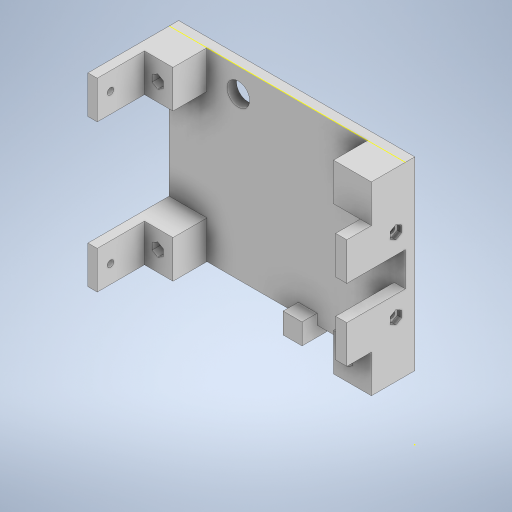
# Autodesk Inventor part: base-prototipo
Saved by Autodesk Inventor 2024.3 (Build 283343000, 343)
## iProperties
Created: 2025-10-16
Part Number: base-prototipo
Material: Genérico
Document SubType Name: Modeling
Designer: julio
Density: 1 g/cm^3
Appearance: Valor por defecto
Author: julio
## iProperties of the stored document Tapadera-prototipo_3DPrint.ipt
Created: 2025-10-16
Part Number: Tapadera-prototipo_3DPrint
Material: Genérico
Document SubType Name: Modeling
Designer: julio
Density: 1 g/cm^3
Appearance: Valor por defecto
Author: julio
Autodesk Inventor part; units mm, degrees
ref_plane "YZ Plane" through (0, 0, 0) normal (1, 0, 0) x (0, 1, 0)
ref_plane "XZ Plane" through (0, 0, 0) normal (0, 1, 0) x (-1, 0, 0)
ref_plane "XY Plane" through (0, 0, 0) normal (0, 0, 1) x (1, 0, 0)
sketch "Boceto1" plane through (0, 0, 0) normal (0, 0, 1) x (1, 0, 0)
  line L0 (-129.8713, 126.9415) -> (-4.8713, 126.9415)
  line L1 (-4.8713, 126.9415) -> (-4.8713, 28.9415)
  line L2 (-4.8713, 28.9415) -> (-129.8713, 28.9415)
  line L3 (-129.8713, 28.9415) -> (-129.8713, 126.9415)
  point P0 (0, 0)
  dimension "d0" = 98
  dimension "d1" = 125
  constraints: 8 end point, 2 parallel, 1 horizontal, 1 perpendicular
  measures "d0" distance of L0.end L1.end
  measures "d1" distance of L0.start L0.end
extrude "Extrusión1" add sketch "Boceto1" along normal blind 5
sketch "Boceto2" plane through (0, 0, 5) normal (0, 0, 1) x (1, 0, 0)
  line L0 (-4.8713, 126.9415) -> (-129.8713, 126.9415) projected
  point P0 (0, 0)
sketch "Boceto3" plane through (0, 0, 5) normal (0, 0, 1) x (1, 0, 0)
  line L0 (-129.8713, 126.9415) -> (-129.8713, 28.9415) projected
  line L1 (-124.9455, 121.4415) -> (-10.7713, 121.4415) construction
  line L2 (-10.7713, 121.4415) -> (-10.7713, 34.4465) construction
  line L3 (-10.7713, 34.4465) -> (-124.9455, 34.4465) construction
  line L4 (-124.9455, 34.4465) -> (-124.9455, 121.4415) construction
  line L5 (-4.8713, 28.9415) -> (-4.8713, 126.9415) projected
  line L6 (-4.8713, 126.9415) -> (-129.8713, 126.9415) projected
  line L7 (-129.8713, 28.9415) -> (-4.8713, 28.9415) projected
  line L8 (-129.8713, 126.9415) -> (-109.8713, 126.9415)
  line L9 (-109.8713, 126.9415) -> (-109.8713, 106.9415)
  line L10 (-109.8713, 106.9415) -> (-129.8713, 106.9415)
  line L11 (-129.8713, 106.9415) -> (-129.8713, 126.9415)
  line L12 (-129.8713, 28.9415) -> (-109.8713, 28.9415)
  line L13 (-109.8713, 28.9415) -> (-109.8713, 48.9415)
  line L14 (-109.8713, 48.9415) -> (-129.8713, 48.9415)
  line L15 (-129.8713, 48.9415) -> (-129.8713, 28.9415)
  line L16 (-4.8713, 28.9415) -> (-24.8713, 28.9415)
  line L17 (-24.8713, 28.9415) -> (-24.8713, 48.9415)
  line L18 (-24.8713, 48.9415) -> (-4.8713, 48.9415)
  line L19 (-4.8713, 48.9415) -> (-4.8713, 28.9415)
  line L20 (-4.8713, 126.9415) -> (-24.8713, 126.9415)
  line L21 (-24.8713, 126.9415) -> (-24.8713, 106.9415)
  line L22 (-24.8713, 106.9415) -> (-4.8713, 106.9415)
  line L23 (-4.8713, 106.9415) -> (-4.8713, 126.9415)
  point P0 (0, 0)
  point P1 (-109.8713, 28.9415)
  point P2 (-4.8713, 106.9415)
  dimension "d58" = 86.995
  dimension "d62" = 114.1741
  dimension "d67" = 5.9
  dimension "d68" = 4.9259
  dimension "d70" = 5.5
  dimension "d71" = 5.505
  dimension "d86" = 20
  dimension "d87" = 20
  dimension "d88" = 20
  dimension "d89" = 20
  dimension "d90" = 20
  dimension "d91" = 20
  dimension "d92" = 20
  dimension "d93" = 20
  constraints: 32 end point, 8 parallel, 4 horizontal, 4 perpendicular, 1 coincident, 2 other
  measures "d58" distance between parallel lines of L3 L1
  measures "d62" distance between parallel lines of L2 L4
  measures "d67" distance between parallel lines of L5 L2
  measures "d68" distance between parallel lines of L4 L0
  measures "d70" distance between parallel lines of L1 L6
  measures "d71" distance between parallel lines of L7 L3
  measures "d86" distance of L8.end L9.end
  measures "d87" distance of L9.end L10.end
  measures "d88" distance of L12.end L13.end
  measures "d89" distance of L13.end L14.end
  measures "d90" distance of L17.end L18.end
  measures "d91" distance of L16.end L17.end
  measures "d92" distance of L20.end L21.end
  measures "d93" distance of L21.end L22.end
extrude "Extrusión2" add sketch "Boceto3" along normal blind 18 contours L6 L9 L10 L0 | L14 L13 L7 L0 | L6 L5 L22 L21 | L17 L18 L5 L7
sketch "Boceto4" plane through (0, 0, 23) normal (0, 0, 1) x (1, 0, 0)
  line L0 (-124.9585, 121.4415) -> (-10.7843, 121.4415) construction
  line L1 (-10.7843, 121.4415) -> (-10.7843, 34.4465) construction
  line L2 (-10.7843, 34.4465) -> (-124.9585, 34.4465) construction
  line L3 (-124.9585, 34.4465) -> (-124.9585, 121.4415) construction
  line L4 (-4.8713, 48.9415) -> (-4.8713, 106.9415) projected
  line L5 (-24.8713, 126.9415) -> (-109.8713, 126.9415) projected
  line L6 (-109.8713, 28.9415) -> (-24.8713, 28.9415) projected
  line L7 (-129.8713, 106.9415) -> (-129.8713, 48.9415) projected
  line L8 (-129.8713, 106.9415) -> (-109.8713, 106.9415) projected
  line L9 (-129.8713, 126.9415) -> (-124.9585, 126.9415)
  line L10 (-124.9585, 126.9415) -> (-124.9585, 106.9415)
  line L11 (-124.9585, 106.9415) -> (-129.8713, 106.9415)
  line L12 (-129.8713, 106.9415) -> (-129.8713, 126.9415)
  line L13 (-124.9585, 28.9415) -> (-129.8713, 28.9415)
  line L14 (-129.8713, 28.9415) -> (-129.8713, 48.9415)
  line L15 (-129.8713, 48.9415) -> (-124.9585, 48.9415)
  line L16 (-124.9585, 48.9415) -> (-124.9585, 28.9415)
  line L17 (-4.8713, 28.9415) -> (-4.8713, 126.9415) projected
  point P0 (0, 0)
  point P1 (-10.7843, 48.9415)
  dimension "d105" = 5.5
  dimension "d106" = 5.505
  dimension "d108" = 5.913
  dimension "d109" = 4.9129
  dimension "d111" = 20
  constraints: 16 end point, 5 point on line, 4 parallel, 2 horizontal, 2 perpendicular, 2 other
  measures "d105" distance between parallel lines of L5 L0
  measures "d106" distance between parallel lines of L2 L6
  measures "d108" distance between parallel lines of L4 L1
  measures "d109" distance between parallel lines of L7 L3
  measures "d111" distance between parallel lines of L8 L9
extrude "Extrusión3" add sketch "Boceto4" along normal blind 25
sketch "Boceto5" plane through (0, 0, 5) normal (0, 0, 1) x (1, 0, 0)
  line L0 (-4.8713, 48.9415) -> (-4.8713, 106.9415) projected
  line L1 (-4.8713, 48.9415) -> (-10.7843, 48.9415)
  line L2 (-10.7843, 48.9415) -> (-10.7843, 68.9415)
  line L3 (-10.7843, 68.9415) -> (-4.8713, 68.9415)
  line L4 (-4.8713, 68.9415) -> (-4.8713, 48.9415)
  line L5 (-4.8713, 106.9415) -> (-24.8713, 106.9415) projected
  line L6 (-4.8713, 106.9415) -> (-10.7843, 106.9415)
  line L7 (-10.7843, 106.9415) -> (-10.7843, 86.9415)
  line L8 (-10.7843, 86.9415) -> (-4.8713, 86.9415)
  line L9 (-4.8713, 86.9415) -> (-4.8713, 106.9415)
  point P0 (0, 0)
  dimension "d120" = 20
  dimension "d121" = 5.913
  dimension "d122" = 20
  constraints: 16 end point, 4 parallel, 2 horizontal, 2 perpendicular, 1 point on line
  measures "d120" distance of L6.end L7.end
  measures "d121" distance of L7.end L8.end
  measures "d122" distance of L1.end L2.end
extrude "Extrusión4" add sketch "Boceto5" along normal blind 31
sketch "Boceto6" plane through (0, 0, 5) normal (0, 0, 1) x (1, 0, 0)
  line L0 (-10.7843, 120.6745) -> (-10.7843, 34.4415) construction
  line L1 (-123.9583, 34.4415) -> (-123.9583, 120.6745) construction
  line L2 (-10.7843, 34.4415) -> (-123.9583, 34.4415) construction
  line L3 (-123.9583, 120.6745) -> (-10.7843, 120.6745) construction
  line L4 (-4.8713, 68.9415) -> (-4.8713, 86.9415) projected
  line L5 (-129.8713, 106.9415) -> (-129.8713, 48.9415) projected
  line L6 (-109.8713, 28.9415) -> (-24.8713, 28.9415) projected
  line L7 (-24.8713, 126.9415) -> (-109.8713, 126.9415) projected
  line L8 (-61.5713, 34.4415) -> (-51.5713, 34.4415)
  line L9 (-51.5713, 34.4415) -> (-51.5713, 28.9415)
  line L10 (-51.5713, 28.9415) -> (-61.5713, 28.9415)
  line L11 (-61.5713, 28.9415) -> (-61.5713, 34.4415)
  line L12 (-4.8713, 28.9415) -> (-4.8713, 48.9415) projected
  line L13 (-129.8713, 48.9415) -> (-129.8713, 28.9415) projected
  point P0 (0, 0)
  point P1 (-123.9583, 118.8668)
  point P2 (-123.9583, 40.8668)
  point P3 (-10.7843, 60.8668)
  point P4 (-51.5713, 31.6915)
  point P5 (-61.5713, 28.9415)
  dimension "d130" = 5.913
  dimension "d131" = 5.913
  dimension "d132" = 5.5
  dimension "d133" = 6.267
  dimension "d135" = 10
  dimension "d136" = 46.7
  dimension "d137" = 68.3
  constraints: 8 end point, 5 point on line, 2 parallel, 1 horizontal, 1 midpoint, 1 perpendicular, 2 other
  measures "d130" distance between parallel lines of L4 L0
  measures "d131" distance between parallel lines of L5 L1
  measures "d132" distance between parallel lines of L6 L2
  measures "d133" distance between parallel lines of L7 L3
  measures "d135" distance from line of point (-51.571, 31.692) L11
  measures "d136" distance between parallel lines of L12 L9
  measures "d137" distance between parallel lines of L13 L11
extrude "Extrusión5" add sketch "Boceto6" along normal blind 8
sketch "Boceto7" plane through (-129.8713, 28.9415, 0) normal (0, -1, 0) x (1, 0, 0)
  line L0 (68.3, 5) -> (68.3, 13) projected
  line L1 (68.3, 13) -> (78.3, 13)
  line L2 (78.3, 13) -> (78.3, 0)
  line L3 (78.3, 0) -> (68.3, 0)
  line L4 (68.3, 0) -> (68.3, 13)
  line L5 (0, 0) -> (125, 0) projected
  point P0 (129.8713, 0)
  point P1 (78.3, 5)
  constraints: 8 end point, 3 point on line, 2 parallel, 1 horizontal, 1 perpendicular
extrude "Extrusión6" add sketch "Boceto7" along normal blind 5.5
sketch "Boceto8" plane through (-4.8713, 28.9415, 0) normal (1, 0, 0) x (0, 0, -1)
  line L0 (-7, 31.25) -> (-7, 27.75)
  line L1 (-7, 27.75) -> (-10.0311, 26)
  line L2 (-10.0311, 26) -> (-13.0622, 27.75)
  line L3 (-13.0622, 27.75) -> (-13.0622, 31.25)
  line L4 (-13.0622, 31.25) -> (-10.0311, 33)
  line L5 (-10.0311, 33) -> (-7, 31.25)
  line L6 (0, 0) -> (0, 98) projected
  line L7 (-5, 40) -> (-36, 40) projected
  line L8 (-5, 58) -> (-36, 58) projected
  line L9 (-7, 70.25) -> (-7, 66.75)
  line L10 (-7, 66.75) -> (-10.0311, 65)
  line L11 (-10.0311, 65) -> (-13.0622, 66.75)
  line L12 (-13.0622, 66.75) -> (-13.0622, 70.25)
  line L13 (-13.0622, 70.25) -> (-10.0311, 72)
  line L14 (-10.0311, 72) -> (-7, 70.25)
  point P0 (0, -28.9415)
  point P1 (-10.0311, 29.5)
  point P2 (-7, 29.5)
  point P3 (-10.0311, 68.5)
  point P4 (-7, 68.5)
  dimension "d149" = 3.5
  dimension "d151" = 7
  dimension "d153" = 7
  dimension "d156" = 3.5
  dimension "d157" = 7
  dimension "d158" = 7
  constraints: 24 end point, 2 midpoint, 1 parallel, 26 other
  measures "d149" distance of L2.end L3.end
  measures "d151" distance from line of L7 L4.end
  measures "d153" distance from line of L6 point (-7, 29.5)
  measures "d156" distance of L11.end L12.end
  measures "d157" distance from line of L8 L10.end
  measures "d158" distance from line of L6 point (-7, 68.5)
extrude "Extrusión7" cut sketch "Boceto8" against normal blind 2.3
sketch "Boceto9" plane through (0, 0, 5) normal (0, 0, 1) x (1, 0, 0)
  point P0 (0, 0)
sketch "Boceto10" plane through (-7.1713, 28.9415, 0) normal (1, 0, 0) x (0, 0, -1)
  circle A0 centre (-10.0311, 29.5) radius 1.75
  line L0 (-13.0622, 27.75) -> (-13.0622, 31.25) projected
  line L1 (-10.0311, 33) -> (-7, 31.25) projected
  line L2 (-7, 31.25) -> (-7, 27.75) projected
  line L3 (-13.0622, 31.25) -> (-10.0311, 33) projected
  line L4 (-7, 27.75) -> (-10.0311, 26) projected
  circle A1 centre (-10.0311, 68.5) radius 1.75
  line L5 (-10.0311, 65) -> (-13.0622, 66.75) projected
  line L6 (-13.0622, 66.75) -> (-13.0622, 70.25) projected
  line L7 (-10.0311, 72) -> (-7, 70.25) projected
  line L8 (-7, 70.25) -> (-7, 66.75) projected
  point P0 (0, -28.9415)
  dimension "d161" = 3.5
  dimension "d162" = 3.5
  dimension "d163" = 3.5
  dimension "d164" = 3.5
  dimension "d165" = 3.5
  dimension "d166" = 3.5
  dimension "d167" = 3.5
  dimension "d168" = 3.5
  dimension "d169" = 3.5
  dimension "d170" = 3.5
  dimension "d171" = 3.5
  constraints: 2 centre point, 2 coincident
  measures "d161" diameter of A0
  measures "d162" distance of point (-13.062, 31.25) A0.centre
  measures "d163" distance of A0.centre L0.start
  measures "d164" distance of L1.end A0.centre
  measures "d165" distance of A0.centre L2.end
  measures "d166" distance of L4.end A0.centre
  measures "d167" distance of L6.end A1.centre
  measures "d168" distance of A1.centre L5.end
  measures "d169" distance of A1.centre L8.end
  measures "d170" distance of L7.end A1.centre
  measures "d171" diameter of A1
extrude "Extrusión8" cut sketch "Boceto10" against normal blind 5
sketch "Boceto11" plane through (-129.8713, 28.9415, 0) normal (-1, 0, 0) x (0, 0, 1)
  line L0 (37.9689, 86.75) -> (37.9689, 90.25)
  line L1 (37.9689, 90.25) -> (41, 92)
  line L2 (41, 92) -> (44.0311, 90.25)
  line L3 (44.0311, 90.25) -> (44.0311, 86.75)
  line L4 (44.0311, 86.75) -> (41, 85)
  line L5 (41, 85) -> (37.9689, 86.75)
  line L6 (37.9689, 7.75) -> (37.9689, 11.25)
  line L7 (37.9689, 11.25) -> (41, 13)
  line L8 (41, 13) -> (44.0311, 11.25)
  line L9 (44.0311, 11.25) -> (44.0311, 7.75)
  line L10 (44.0311, 7.75) -> (41, 6)
  line L11 (41, 6) -> (37.9689, 7.75)
  line L12 (48, 20) -> (48, 0) projected
  line L13 (48, 98) -> (48, 78) projected
  line L14 (5, 78) -> (48, 78) projected
  line L15 (5, 20) -> (48, 20) projected
  point P0 (0, -28.9415)
  point P1 (41, 88.5)
  point P2 (41, 9.5)
  point P3 (48, 10)
  dimension "d174" = 7
  dimension "d175" = 3.5
  dimension "d176" = 7
  dimension "d177" = 3.5
  dimension "d178" = 7
  dimension "d179" = 7
  constraints: 24 end point, 2 parallel, 1 midpoint, 26 other
  measures "d174" distance from line of L14 L4.end
  measures "d175" distance of L8.end L9.end
  measures "d176" distance from line of L15 L7.end
  measures "d177" distance of L2.end L3.end
  measures "d178" horizontal distance of point (48, 10) point (41, 9.5)
  measures "d179" distance from line of L13 point (41, 88.5)
extrude "Extrusión9" cut sketch "Boceto11" against normal blind 2.3
sketch "Boceto12" plane through (-127.5713, 28.9415, 0) normal (-1, 0, 0) x (0, 0, 1)
  circle A0 centre (41, 88.5) radius 1.75
  line L0 (44.0311, 86.75) -> (41, 85) projected
  line L1 (37.9689, 90.25) -> (41, 92) projected
  line L2 (41, 85) -> (37.9689, 86.75) projected
  line L3 (44.0311, 90.25) -> (44.0311, 86.75) projected
  circle A1 centre (41, 9.5) radius 1.75
  line L4 (44.0311, 11.25) -> (44.0311, 7.75) projected
  line L5 (37.9689, 11.25) -> (41, 13) projected
  point P0 (0, -28.9415)
  dimension "d182" = 3.5
  dimension "d184" = 3.5
  dimension "d187" = 3.5
  dimension "d188" = 3.5
  dimension "d189" = 3.5
  dimension "d190" = 3.5
  dimension "d191" = 3.5
  dimension "d192" = 3.5
  constraints: 2 centre point, 1 coincident
  measures "d182" diameter of A0
  measures "d184" distance of L3.start A0.centre
  measures "d187" distance of L2.end A0.centre
  measures "d188" distance of L1.start A0.centre
  measures "d189" diameter of A1
  measures "d190" distance of point (44.031, 7.75) A1.centre
  measures "d191" distance of A1.centre L4.start
  measures "d192" distance of A1.centre L5.start
extrude "Extrusión10" cut sketch "Boceto12" against normal blind 5
sketch "Boceto13" plane through (0, 0, 23) normal (0, 0, 1) x (1, 0, 0)
  line L0 (-20.8713, 37.6915) -> (-20.8713, 41.1915)
  line L1 (-20.8713, 41.1915) -> (-17.8403, 42.9415)
  line L2 (-17.8403, 42.9415) -> (-14.8092, 41.1915)
  line L3 (-14.8092, 41.1915) -> (-14.8092, 37.6915)
  line L4 (-14.8092, 37.6915) -> (-17.8403, 35.9415)
  line L5 (-17.8403, 35.9415) -> (-20.8713, 37.6915)
  line L6 (-24.8713, 48.9415) -> (-24.8713, 28.9415) projected
  line L7 (-10.7843, 48.9415) -> (-24.8713, 48.9415) projected
  line L8 (-120.9585, 37.6915) -> (-120.9585, 41.1915)
  line L9 (-120.9585, 41.1915) -> (-117.9274, 42.9415)
  line L10 (-117.9274, 42.9415) -> (-114.8963, 41.1915)
  line L11 (-114.8963, 41.1915) -> (-114.8963, 37.6915)
  line L12 (-114.8963, 37.6915) -> (-117.9274, 35.9415)
  line L13 (-117.9274, 35.9415) -> (-120.9585, 37.6915)
  line L14 (-124.9585, 28.9415) -> (-124.9585, 48.9415) projected
  line L15 (-109.8713, 48.9415) -> (-124.9585, 48.9415) projected
  line L16 (-120.9585, 114.6915) -> (-120.9585, 118.1915)
  line L17 (-120.9585, 118.1915) -> (-117.9274, 119.9415)
  line L18 (-117.9274, 119.9415) -> (-114.8963, 118.1915)
  line L19 (-114.8963, 118.1915) -> (-114.8963, 114.6915)
  line L20 (-114.8963, 114.6915) -> (-117.9274, 112.9415)
  line L21 (-117.9274, 112.9415) -> (-120.9585, 114.6915)
  line L22 (-124.9585, 106.9415) -> (-124.9585, 126.9415) projected
  line L23 (-124.9585, 106.9415) -> (-109.8713, 106.9415) projected
  line L24 (-13.0065, 121.4993) -> (-13.0065, 35.2663) construction
  line L25 (-126.1805, 35.2663) -> (-126.1805, 121.4993) construction
  line L26 (-13.0065, 35.2663) -> (-126.1805, 35.2663) construction
  line L27 (-126.1805, 121.4993) -> (-13.0065, 121.4993) construction
  point P0 (0, 0)
  point P1 (-17.8403, 39.4415)
  point P2 (-20.8713, 39.4415)
  point P3 (-117.9274, 39.4415)
  point P4 (-120.9585, 39.4415)
  point P5 (-117.9274, 116.4415)
  point P6 (-13.0065, 61.6917)
  point P7 (-126.1805, 119.6917)
  point P8 (-126.1805, 41.6917)
  point P9 (-63.7935, 35.2663)
  dimension "d195" = 3.5
  dimension "d196" = 6
  dimension "d197" = 4
  dimension "d198" = 6
  dimension "d199" = 4
  dimension "d200" = 6
  dimension "d201" = 4
  dimension "d202" = 3.5
  dimension "d203" = 3.5
  constraints: 36 end point, 4 point on line, 3 parallel, 2 midpoint, 41 other
  measures "d195" distance of L2.end L3.end
  measures "d196" distance from line of L7 L1.end
  measures "d197" distance from line of L6 point (-20.871, 39.442)
  measures "d198" distance from line of L15 L9.end
  measures "d199" distance from line of L14 point (-120.958, 39.442)
  measures "d200" distance from line of L23 L20.end
  measures "d201" distance between parallel lines of L22 L16
  measures "d202" distance of L18.end L19.end
  measures "d203" distance of L10.end L11.end
extrude "Extrusión11" cut sketch "Boceto13" against normal blind 6
sketch "Boceto17" plane through (0, 0, 23) normal (0, 0, 1) x (1, 0, 0)
  circle A0 centre (-17.8403, 39.4415) radius 2
  line L0 (-14.8092, 41.1915) -> (-14.8092, 37.6915) projected
  line L1 (-14.8092, 41.1915) -> (-14.8092, 37.6915) projected
  line L2 (-20.8713, 41.1915) -> (-17.8403, 42.9415) projected
  circle A1 centre (-117.9274, 39.4415) radius 2
  line L3 (-117.9274, 42.9415) -> (-114.8963, 41.1915) projected
  line L4 (-120.9585, 37.6915) -> (-120.9585, 41.1915) projected
  line L5 (-114.8963, 37.6915) -> (-117.9274, 35.9415) projected
  circle A2 centre (-117.9274, 116.4415) radius 2
  line L6 (-117.9274, 119.9415) -> (-114.8963, 118.1915) projected
  line L7 (-120.9585, 114.6915) -> (-120.9585, 118.1915) projected
  point P0 (0, 0)
  point P1 (-20.8713, 37.6915)
  point P2 (-114.8963, 114.6915)
  dimension "d236" = 4
  dimension "d238" = 3.5
  dimension "d239" = 3.5
  dimension "d240" = 4
  dimension "d241" = 3.5
  dimension "d243" = 3.5
  dimension "d244" = 4
  dimension "d245" = 3.5
  dimension "d246" = 3.5
  dimension "d247" = 3.5
  dimension "d248" = 3.5
  dimension "d249" = 3.5
  constraints: 3 centre point, 2 coincident
  measures "d236" diameter of A0
  measures "d238" distance of L2.start A0.centre
  measures "d239" distance of point (-14.809, 37.692) A0.centre
  measures "d240" diameter of A1
  measures "d241" distance of L3.end A1.centre
  measures "d243" distance of L4.end A1.centre
  measures "d244" diameter of A2
  measures "d245" distance of A2.centre L6.end
  measures "d246" distance of L7.start A2.centre
  measures "d247" distance of A2.centre point (-114.896, 114.692)
  measures "d248" distance of L7.end A2.centre
  measures "d249" distance of L4.start A1.centre
extrude "Extrusión15" cut sketch "Boceto17" against normal blind 15
sketch "Boceto18" plane through (0, 0, 5) normal (0, 0, 1) x (1, 0, 0)
  line L0 (125.8009, 116.9426) -> (125.8009, 30.6207) construction
  line L1 (12.5101, 30.6207) -> (12.5101, 116.9426) construction
  line L2 (125.8009, 30.6207) -> (12.5101, 30.6207) construction
  line L3 (12.5101, 116.9426) -> (125.8009, 116.9426) construction
  line L4 (-10.9427, 120.5005) -> (-10.9427, 34.2675) construction
  line L5 (-124.1167, 34.2675) -> (-124.1167, 120.5005) construction
  line L6 (-10.9427, 34.2675) -> (-124.1167, 34.2675) construction
  line L7 (-124.1167, 120.5005) -> (-10.9427, 120.5005) construction
  circle A0 centre (-93.2833, 114.0005) radius 6
  line L8 (-109.8713, 106.9415) -> (-109.8713, 126.9415) projected
  line L9 (-100.2833, 119.5538) -> (-100.2833, 109.0268)
  line L10 (-129.8713, 106.9415) -> (-129.8713, 48.9415) projected
  line L11 (-24.8713, 126.9415) -> (-109.8713, 126.9415) projected
  point P0 (0, 0)
  point P1 (-11.7474, -20.2697)
  point P2 (-124.9214, 37.7303)
  point P3 (-124.9214, -40.2697)
  point P4 (-146.9688, 35.7152)
  point P5 (-10.185, 48.671)
  point P6 (-123.359, 106.671)
  point P7 (-123.359, 28.671)
  point P8 (-56.0563, 34.9687)
  point P9 (125.8009, 4.0884)
  point P10 (12.5101, 62.0884)
  point P11 (12.5101, -15.9116)
  point P12 (-197.4234, 30.6207)
  point P13 (-10.9427, 45.9824)
  point P14 (-124.1167, 103.9824)
  point P15 (-124.1167, 25.9824)
  point P16 (-58.9128, 34.2675)
  point P17 (-95.5526, 120.5005)
  point P18 (-100.2833, 114.2903)
  dimension "d283" = 12
  dimension "d299" = 9.5881
  dimension "d301" = 6.5
  dimension "d303" = 7
  dimension "d305" = 5.7546
  dimension "d307" = 6.441
  constraints: 9 point on line, 2 end point, 1 centre point, 1 midpoint, 1 vertical, 4 other
  measures "d283" diameter of A0
  measures "d299" distance from line of L8 point (-100.283, 114.29)
  measures "d301" distance from line of A0.centre L7
  measures "d303" distance from line of L9 A0.centre
  measures "d305" distance between parallel lines of L10 L5
  measures "d307" distance between parallel lines of L11 L7
extrude "Extrusión16" cut sketch "Boceto18" against normal blind 10
